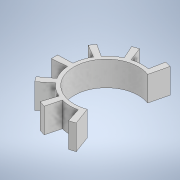
# Autodesk Inventor part: pneunet_approximate_test_second_bend
Saved by Autodesk Inventor 2021 (Build 250183000, 183)
## iProperties
Created: 2021-03-25
Part Number: pneunet_approximate_test_second_bend
Material: Generic
Document SubType Name: Modeling
Designer: Charlie
Density: 1 g/cm^3
Appearance: Default
Author: Charlie
Autodesk Inventor part; units mm, degrees
ref_plane "YZ Plane" through (0, 0, 0) normal (1, 0, 0) x (0, 1, 0)
ref_plane "XZ Plane" through (0, 0, 0) normal (0, 1, 0) x (-1, 0, 0)
ref_plane "XY Plane" through (0, 0, 0) normal (0, 0, 1) x (1, 0, 0)
sketch "Sketch1" plane through (0, 0, 0) normal (0, 1, 0) x (-1, 0, 0)
  line L0 (-141.9954, -89.0732) -> (-156.9954, -89.0732) construction
  line L1 (-141.9954, -169.2741) -> (-141.9954, -89.0732) construction
  line L2 (-141.9954, -89.0732) -> (-156.9954, -173.6661) construction
  line L3 (-141.9954, -89.0732) -> (-141.9954, -94.0732) construction
  line L4 (-141.9954, -104.0732) -> (-153.9954, -104.0732) construction
  line L5 (-153.9954, -104.0732) -> (-153.9954, -94.0732) construction
  line L6 (-153.9954, -94.0732) -> (-141.9954, -94.0732) construction
  line L7 (-141.9954, -120.0732) -> (-153.9954, -120.0732) construction
  line L8 (-153.9954, -120.0732) -> (-153.9954, -110.0732) construction
  line L9 (-153.9954, -110.0732) -> (-141.9954, -110.0732) construction
  line L10 (-141.9954, -136.0732) -> (-153.9954, -136.0732) construction
  line L11 (-153.9954, -136.0732) -> (-153.9954, -126.0732) construction
  line L12 (-153.9954, -126.0732) -> (-141.9954, -126.0732) construction
  line L13 (-141.9954, -152.0732) -> (-153.9954, -152.0732) construction
  line L14 (-153.9954, -152.0732) -> (-153.9954, -142.0732) construction
  line L15 (-153.9954, -142.0732) -> (-141.9954, -142.0732) construction
  line L16 (-141.9954, -168.0732) -> (-153.9954, -168.0732) construction
  line L17 (-153.9954, -168.0732) -> (-153.9954, -158.0732) construction
  line L18 (-153.9954, -158.0732) -> (-141.9954, -158.0732) construction
  line L19 (-141.9954, -184.0732) -> (-153.9954, -184.0732) construction
  line L20 (-153.9954, -184.0732) -> (-153.9954, -174.0732) construction
  line L21 (-153.9954, -174.0732) -> (-141.9954, -174.0732) construction
  line L22 (-141.9954, -104.0732) -> (-141.9954, -110.0732) construction
  line L23 (-141.9954, -120.0732) -> (-141.9954, -126.0732) construction
  line L24 (-141.9954, -136.0732) -> (-141.9954, -142.0732) construction
  line L25 (-141.9954, -152.0732) -> (-141.9954, -158.0732) construction
  arc A0 (-115.1624, -166.0515) -> (-115.1624, -81.4587) centre (-143.2186, -123.7551) ccw
  line L26 (-156.9954, -89.0732) -> (-156.9954, -189.0732) construction
  line L27 (-156.9954, -189.0732) -> (-141.9954, -189.0732) construction
  line L28 (-141.9954, -189.0732) -> (-141.9954, -184.0732) construction
  line L29 (-106.8702, -68.959) -> (-115.1624, -81.4587)
  line L30 (-106.8702, -68.959) -> (-102.7037, -71.7231)
  line L31 (-109.4661, -81.9168) -> (-102.7037, -71.7231)
  line L32 (-98.2749, -94.2637) -> (-88.7156, -86.6308)
  line L33 (-91.8355, -82.7236) -> (-88.7156, -86.6308)
  line L34 (-91.8355, -82.7236) -> (-103.5572, -92.0831)
  line L35 (-91.4027, -109.4447) -> (-79.9652, -105.1061)
  line L36 (-81.7385, -100.4311) -> (-79.9652, -105.1061)
  line L37 (-81.7385, -100.4311) -> (-95.7634, -105.7512)
  line L38 (-89.5099, -126.0009) -> (-77.2932, -125.3735)
  line L39 (-77.5496, -120.3801) -> (-77.2932, -125.3735)
  line L40 (-77.5496, -120.3801) -> (-92.5299, -121.1494)
  line L41 (-92.7783, -142.3413) -> (-80.9564, -145.4853)
  line L42 (-79.6713, -140.6533) -> (-80.9564, -145.4853)
  line L43 (-79.6713, -140.6533) -> (-94.1674, -136.798)
  line L44 (-100.8939, -156.8955) -> (-90.6029, -163.509)
  line L45 (-87.8998, -159.3027) -> (-90.6029, -163.509)
  line L46 (-87.8998, -159.3027) -> (-100.5186, -151.1932)
  line L47 (-113.0768, -168.2651) -> (-105.3056, -177.7124)
  line L48 (-101.4442, -174.536) -> (-105.3056, -177.7124)
  line L49 (-101.4442, -174.536) -> (-110.9732, -162.9517)
  arc A1 (-113.0768, -168.2651) -> (-113.5041, -78.9587) centre (-143.2186, -123.7551) ccw
  line L50 (-105.3056, -177.7124) -> (-114.9914, -165.9376)
  arc A2 (-8.9885, -24.3841) -> (-8.9885, 24.3841) centre (0, 0) ccw
  arc A3 (-10.0261, -27.1989) -> (-10.0261, 27.1989) centre (0, 0) ccw
  line L51 (0, 0) -> (-10.0261, 27.1989) construction
  line L52 (-8.9885, 24.3841) -> (-14.1801, 38.457)
  line L53 (-14.1801, 38.457) -> (-9.3733, 39.8337)
  line L54 (-9.3733, 39.8337) -> (-4.8541, 25.5307)
  line L55 (6.6962, 25.1105) -> (10.5576, 39.605)
  line L56 (10.5576, 39.605) -> (15.28, 37.9619)
  line L57 (15.28, 37.9619) -> (10.7365, 23.6665)
  line L58 (19.9366, 16.6706) -> (31.4414, 26.2955)
  line L59 (31.4414, 26.2955) -> (34.3555, 22.2325)
  line L60 (34.3555, 22.2325) -> (22.4077, 13.1632)
  line L61 (25.8993, 2.1453) -> (40.8478, 3.3872)
  line L62 (40.8478, 3.3872) -> (40.8899, -1.6126)
  line L63 (40.8899, -1.6126) -> (25.8993, -2.1453)
  line L64 (22.4077, -13.1632) -> (35.3431, -20.7576)
  line L65 (35.3431, -20.7576) -> (32.4978, -24.8691)
  line L66 (32.4978, -24.8691) -> (19.9366, -16.6706)
  line L67 (10.7365, -23.6665) -> (16.9368, -37.3251)
  line L68 (16.9368, -37.3251) -> (12.2428, -39.0473)
  line L69 (12.2428, -39.0473) -> (6.6962, -25.1105)
  line L70 (-4.8541, -25.5307) -> (-7.6521, -40.2674)
  line L71 (-7.6521, -40.2674) -> (-12.4813, -38.9718)
  line L72 (-12.4813, -38.9718) -> (-8.9885, -24.3841)
  point P0 (0, 0)
  point P1 (-141.9954, -129.1737)
  point P2 (-109.0674, -165.2686)
  point P3 (-100.8939, -156.8955)
  point P4 (-97.9949, -152.8151)
  point P5 (-92.7783, -142.3413)
  point P6 (-91.2682, -137.5691)
  point P7 (-89.5099, -126.0009)
  point P8 (-89.5338, -120.9955)
  point P9 (-91.4027, -109.4447)
  point P10 (-92.9584, -104.6872)
  point P11 (-98.2749, -94.2637)
  point P12 (-101.2129, -90.2112)
  point P13 (-115.1624, -81.4587)
  point P14 (7.4685, 28.0094)
  point P15 (-5.7636, 28.4093)
  point P16 (-5.4137, -28.478)
  point P17 (7.8125, -27.9154)
  point P18 (11.9765, -26.3982)
  point P19 (22.4646, -18.3206)
  point P20 (24.9948, -14.6821)
  point P21 (28.9163, -2.0381)
  point P22 (28.889, 2.3936)
  point P23 (24.8123, 14.9885)
  point P24 (22.2376, 18.5956)
  point P25 (11.6509, 26.5436)
  dimension "d4" = 5
  dimension "d5" = 10
  dimension "d6" = 12
  dimension "d9" = 16
  dimension "d14" = 10
  dimension "d19" = 100
  dimension "d20" = 3
  dimension "d25" = 5
  dimension "d28" = 107
  dimension "d30" = 17.833
  dimension "d31" = 50.7557
  dimension "d32" = 100
  dimension "d33" = 25.988
  dimension "d35" = 3
  dimension "d36" = 15
  dimension "d40" = 15
  dimension "d41" = 5
  dimension "d42" = 15
  dimension "d45" = 211
  dimension "d47" = 40.8749
  constraints: 146 end point, 10 point on circle, 4 centre point, 4 equal length, 3 perpendicular, 2 point on line, 2 vertical, 1 coincident, 1 horizontal, 1 midpoint, 121 other
  measures "d4" distance of L0.start L3.end
  measures "d5" distance of L3.end L4.start
  measures "d6" distance of L4.start L4.end
  measures "d9" distance of L4.start L7.start
  measures "d14" distance of L13.end L14.end
  measures "d19" distance of L0.end L26.end
  measures "d20" distance between parallel lines of L26 L20
  measures "d25" distance of L29.start L30.end
  measures "d30" angle of L40 L35
  measures "d31" radius of A0
  measures "d33" radius of A2
  measures "d35" radial gap between concentric circles of A2 A3
  measures "d36" distance of L0.start L0.end
  measures "d40" distance of L52.start L52.end
  measures "d41" distance of L52.end L53.end
  measures "d42" distance of L53.end L54.end
  measures "d47" distance from line of L65 L51.start
extrude "Extrusion1" add sketch "Sketch1" along normal blind 20 contours A2 L70 A3 L72 | A2 L69 A3 L70 | A3 L70 L71 L72 | A2 L67 A3 L69 | A2 L66 A3 L67 | A3 L67 L68 L69 | A2 L64 A3 L66 | A2 L63 A3 L64 | A3 L64 L65 L66 | A2 L61 A3 L63 | A2 L60 A3 L61 | A3 L61 L62 L63 | A2 L58 A3 L60 | A2 L57 A3 L58 | A3 L58 L59 L60 | A2 L55 A3 L57 | A2 L54 A3 L55 | A3 L55 L56 L57 | A2 L52 A3 L54 | A3 L52 L53 L54
body "Solid1"
